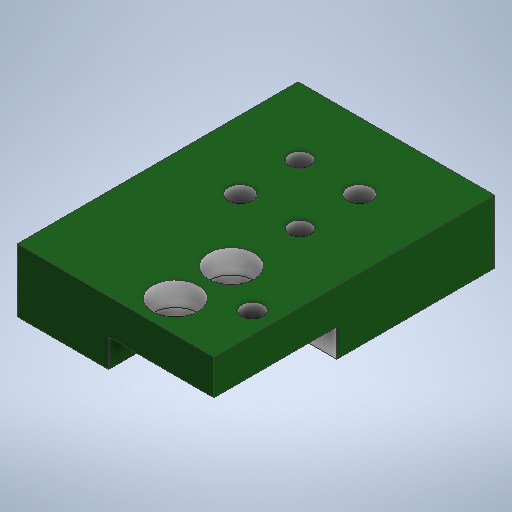
# Autodesk Inventor part: JH_int_Adapterplatte
Saved by Autodesk Inventor 2025.1 (Build 291241000, 241)
## iProperties
Created: 2025-06-17
Part Number: JH_int_Adapterplatte
Material: Generisch
Document SubType Name: Modeling
Designer: Jakob
Density: 1 g/cm^3
Appearance: Vorgabe
Author: Jakob
Autodesk Inventor part; units mm, degrees
ref_plane "YZ Plane" through (0, 0, 0) normal (1, 0, 0) x (0, 1, 0)
ref_plane "XZ Plane" through (0, 0, 0) normal (0, 1, 0) x (-1, 0, 0)
ref_plane "XY Plane" through (0, 0, 0) normal (0, 0, 1) x (1, 0, 0)
sketch "Skizze2" plane through (0, 0, 0) normal (0, 1, 0) x (-1, 0, 0)
  line L0 (14, 0) -> (-14, 0)
  line L1 (-14, 0) -> (-14, -5)
  line L2 (-14, -5) -> (1, -5)
  line L3 (1, -5) -> (1, -9)
  line L4 (1, -9) -> (14, -9)
  line L5 (14, -9) -> (14, 0)
  line L6 (0, -10.8) -> (0, 1.8) projected
  line L7 (19.6, 0) -> (-19.6, 0) projected
  point P0 (0, 0)
  dimension "d4" = 28
  dimension "d5" = 9
  dimension "d6" = 5
  dimension "d8" = 13
  dimension "d9" = 15
  constraints: 12 end point, 3 perpendicular, 2 horizontal, 1 collinear, 1 parallel, 1 other
  measures "d4" distance of L0.start L0.end
  measures "d5" distance of L4.end L0.start
  measures "d6" distance of L0.end L1.end
  measures "d8" distance of L3.end L4.end
  measures "d9" distance of L1.end L2.end
extrude "Extrusion2" add sketch "Skizze2" along normal blind 40
sketch "Skizze4" plane through (0, 40, 0) normal (0, 1, 0) x (1, 0, 0)
  line L0 (14, 5) -> (-1, 5)
  line L1 (-1, 5) -> (-1, 9)
  line L2 (-1, 9) -> (14, 9)
  line L3 (14, 9) -> (14, 5)
  line L4 (14, 5) -> (-1, 9) construction
  line L5 (-1, 5) -> (14, 9) construction
  line L6 (14, 5) -> (-1, 5) projected
  line L7 (-1, 5) -> (-1, 9) projected
  point P0 (0, 0)
  point P1 (6.5, 7)
  constraints: 12 end point, 4 collinear, 2 midpoint, 2 parallel, 1 horizontal, 1 perpendicular
extrude "Extrusion3" add sketch "Skizze4" against normal blind 22.5
sketch "Skizze6" plane through (14, 40, -9) normal (0, 0, -1) x (-1, 0, 0)
  line L0 (14, -48) -> (14, 8) projected
  line L1 (0, 0) -> (28, 0) projected
  point P0 (14, -40)
  point P1 (9.7574, -9.5074)
  point P2 (18.2426, -9.5074)
  point P3 (18.2426, -17.9926)
  point P4 (9.7574, -17.9926)
  dimension "d44" = 8.4853
  dimension "d45" = 8.4853
  dimension "d46" = 9.5074
  dimension "d47" = 17.9926
  constraints: 2 symmetric about line
  measures "d44" distance of point (18.243, -9.507) point (9.757, -9.507)
  measures "d45" distance of point (18.243, -17.993) point (9.757, -17.993)
  measures "d46" distance from line of L1 point (18.243, -9.507)
  measures "d47" distance from line of L1 point (18.243, -17.993)
hole "Bohrung3" at (4.2426, 22.0074, -9) at (-4.2426, 30.4926, -9) direction (0, 0, 1) diameter 3 end through all
hole "Bohrung4" at (4.2426, 30.4926, -9) at (-4.2426, 22.0074, -9) direction (0, 0, 1) diameter 3.4 end through all counterbore diameter 6.5 counterbore depth 3.4 clearance for "Sechskantkopfschraube DIN EN 24017" size "M3" standard "DIN"
sketch "Skizze7" plane through (-14, 0, 0) normal (0, 0, 1) x (1, 0, 0)
  line L0 (-5.6, 0) -> (33.6, 0) projected
  line L1 (28, 0) -> (28, 40) projected
  point P0 (14, 0)
  point P1 (18, 12.5)
  point P2 (18, 4.5)
  point P3 (25, 8.5)
  dimension "d62" = 4.5
  dimension "d63" = 12.5
  dimension "d64" = 8.5
  dimension "d65" = 3
  dimension "d66" = 10
  constraints: 1 vertical alignment
  measures "d62" distance from line of L0 point (18, 4.5)
  measures "d63" distance from line of L0 point (18, 12.5)
  measures "d64" distance from line of L0 point (25, 8.5)
  measures "d65" distance from line of L1 point (25, 8.5)
  measures "d66" distance from line of L1 point (18, 4.5)
hole "Bohrung5" at (4, 12.5, 0) at (4, 4.5, 0) direction (0, 0, -1) diameter 3.4 end through all counterbore diameter 6.5 counterbore depth 3.4 clearance for "Sechskantkopfschraube DIN EN 24017" size "M3" standard "DIN"
hole "Bohrung6" at (11, 8.5, 0) direction (0, 0, -1) diameter 3 end through all
